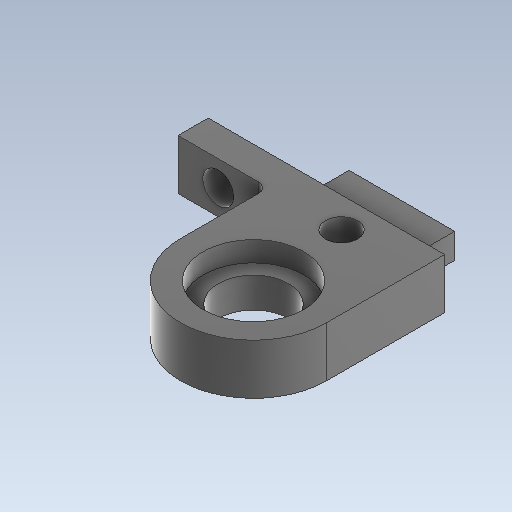
# Autodesk Inventor part: Antenna_frame_01
Saved by Autodesk Inventor 2020.4 (Build 244396000, 396)
## iProperties
Created: 2021-06-09
Part Number: Antenna_frame_01
Material: アセタール樹脂、黒
Document SubType Name: Modeling
Designer: Masato Kubotera
Density: 1.425 g/cm^3
Appearance: 滑らか - 黒
Mass: 1.69286 g
Surface Area: 11.8125 cm^2
Volume: 1.18798 cm^3
Description: POM T5
d0: 3.000 mm
d1: 9.000 mm
d5: 5.000 mm
d8: 1.050 mm
d16: 5.000 mm
d17: 0.00 deg
d18: 3.000 mm
d19: 0.00 deg
d20: 1.000 mm
d21: 4.000 mm
d23: 3.100 mm
d31: 2.500 mm
d32: 0.00 deg
d33: 7.000 mm
d34: 10.000 mm
d38: 4.000 mm
d39: 10.500 mm
d44: 7.250 mm
d45: 7.250 mm
d46: 7.250 mm
d47: 11.750 mm
Author: Masato Kubotera
Title: Antenna_frame_01
Autodesk Inventor part; units mm, degrees
ref_plane "YZ Plane" through (0, 0, 0) normal (1, 0, 0) x (0, 1, 0)
ref_plane "XZ Plane" through (0, 0, 0) normal (0, 1, 0) x (-1, 0, 0)
ref_plane "XY Plane" through (0, 0, 0) normal (0, 0, 1) x (1, 0, 0)
sketch "スケッチ1" plane through (0, 0, 0) normal (0, 0, 1) x (1, 0, 0)
  line L0 (-5.25, -3) -> (-14.25, -3)
  line L1 (-14.25, -3) -> (-14.25, 0)
  line L2 (0, -19) -> (0, 5) construction
  line L3 (-5.25, 2.1) -> (-5.25, 5)
  line L4 (-5.25, 5) -> (5.25, 5)
  arc A0 (-5.25, 0) -> (-5.25, 2.1) centre (-5.25, 1.05) ccw
  line L5 (-14.25, 0) -> (-5.25, 0)
  line L6 (5.25, 2.1) -> (5.25, 5)
  arc A1 (5.25, 2.1) -> (5.25, 0) centre (5.25, 1.05) ccw
  line L7 (-5.25, 0) -> (5.25, 0)
  line L8 (5.25, 0) -> (9.25, 0)
  line L9 (9.25, 0) -> (9.25, -19)
  circle A2 centre (2, -11.75) radius 3.5
  circle A3 centre (2, -11.75) radius 5
  line L10 (-5.25, -19) -> (9.25, -19)
  line L11 (-5.25, -3) -> (-5.25, -19)
  circle A4 centre (2, -3) radius 1.6
  line L12 (2, 0) -> (2, -19) construction
  point P0 (0, 0)
  dimension "d0" = 3
  dimension "d1" = 9
  dimension "d5" = 5
  dimension "d8" = 1.05
  dimension "d33" = 7
  dimension "d34" = 10
  dimension "d38" = 4
  dimension "d39" = 10.5
  dimension "d44" = 7.25
  dimension "d45" = 7.25
  dimension "d47" = 11.75
  dimension "d48" = 3.2
  dimension "d50" = 3
  dimension "d51" = 8.75
  constraints: 26 end point, 8 point on line, 5 centre point, 4 horizontal, 4 perpendicular, 4 point on circle, 4 symmetric about line, 3 midpoint, 2 vertical, 1 coincident, 1 tangent, 1 other
  measures "d0" distance of L0.end L1.end
  measures "d1" distance of L0.start L0.end
  measures "d5" distance of L5.end L3.end
  measures "d8" radius of A0
  measures "d33" diameter of A2
  measures "d34" diameter of A3
  measures "d38" distance between parallel lines of L9 L6
  measures "d39" distance of L3.end L4.end
  measures "d44" distance from line of L9 A2.centre
  measures "d45" distance from line of L10 A2.centre
  measures "d47" distance from line of A2.centre L8
  measures "d48" diameter of A4
  measures "d50" distance of A4.centre L12.start
  measures "d51" distance of A2.centre A4.centre
extrude "押し出し1" add sketch "スケッチ1" along normal blind 5 contours L0 L1 L5 L7 L8 L9 L10 L11
extrude "押し出し2" add sketch "スケッチ1" along normal blind 3 contours A3
fillet "フィレット1" radius 1 1 edges at (-5.25, -3, 2.5)
sketch "スケッチ2" plane through (-14.25, -3, 0) normal (0, -1, 0) x (1, 0, 0)
  line L0 (0, 0) -> (0, 5) projected
  line L1 (0, 2.5) -> (8, 2.5) construction
  line L2 (8, 5) -> (8, 0) projected
  point P0 (14.25, 0)
  point P1 (4, 2.5)
  dimension "d21" = 4
  constraints: 3 midpoint, 2 end point
  measures "d21" distance from line of L0 point (4, 2.5)
hole "穴1" at (-10.25, -3, 2.5) direction (0, 1, 0) diameter 3.1 end through all
extrude "押し出し3" add sketch "スケッチ1" along normal blind 2.5 contours A0 L3 L4 L6 A1 L7
fillet "フィレット2" radius 7.25 2 edges at (-5.25, -19, 2.5) (9.25, -19, 2.5)
equation "\"d45\" = d44"
equation "\"d46\" = d44"
